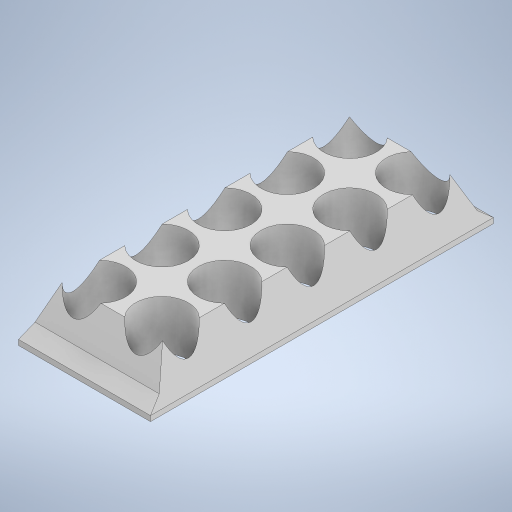
# Autodesk Inventor part: tray
Saved by Autodesk Inventor 2023 (Build 270158000, 158)
## iProperties
Created: 2023-01-16
Part Number: tray
Material: Generic
Document SubType Name: Modeling
Designer: Steven
Density: 1 g/cm^3
Appearance: Default
Author: Steven
Autodesk Inventor part; units mm, degrees
ref_plane "YZ Plane" through (0, 0, 0) normal (1, 0, 0) x (0, 1, 0)
ref_plane "XZ Plane" through (0, 0, 0) normal (0, 1, 0) x (-1, 0, 0)
ref_plane "XY Plane" through (0, 0, 0) normal (0, 0, 1) x (1, 0, 0)
sketch "Sketch1" plane through (0, 0, 0) normal (1, 0, 0) x (0, 1, 0)
  line L0 (0, 520) -> (0, 0)
  line L1 (144.6571, 260) -> (0, 260) construction
  line L2 (0, 0) -> (8, 0)
  line L3 (8, 0) -> (24.0697, 19.1511)
  line L4 (24.0697, 19.1511) -> (75, 42.9003)
  line L5 (0, 520) -> (8, 520)
  line L6 (8, 520) -> (24.0697, 500.8489)
  line L7 (24.0697, 500.8489) -> (75, 477.0997)
  line L8 (75, 477.0997) -> (75, 42.9003)
  dimension "d2" = 520
  dimension "d4" = 8
  dimension "d5" = 130
  dimension "d7" = 25
  dimension "d8" = 260
  dimension "d9" = 115
  dimension "d10" = 75
  constraints: 18 end point, 3 symmetric about line, 1 horizontal, 1 midpoint, 1 vertical
  measures "d2" distance of L0.start L0.end
  measures "d4" distance of L0.end L2.end
  measures "d5" angle of L2 L3
  measures "d7" distance of L2.end L3.end
  measures "d8" distance from line of L0.start L1
  measures "d9" angle of L4 L8
  measures "d10" distance from line of L0 L4.end
extrude "Extrusion1" add sketch "Sketch1" against normal blind 200
sketch "Sketch3" plane through (0, 0, 0) normal (0, 0, -1) x (-1, 0, 0)
  line L0 (0, 8) -> (0, 24.0697) projected
  line L1 (0, 8) -> (24.386, 75)
  line L2 (0, 75) -> (0, 8)
  line L3 (0, 24.0697) -> (0, 75) projected
  line L4 (100, 8) -> (100, 96) construction
  line L5 (200, 8) -> (175.614, 75)
  line L6 (200, 75) -> (200, 8)
  line L7 (0, 75) -> (24.386, 75)
  line L8 (0, 75) -> (200, 75) projected
  line L9 (175.614, 75) -> (200, 75)
  point P0 (0, 0)
  dimension "d13" = 20
  dimension "d14" = 20
  constraints: 14 end point, 2 horizontal, 1 collinear, 1 symmetric about line, 1 other
  measures "d13" angle of L2 L1
  measures "d14" angle of L6 L5
extrude "Extrusion2" cut sketch "Sketch3" against normal through all
sketch "Sketch4" plane through (-175.614, 75, 477.0997) normal (0, 1, 0) x (1, 0, 0)
  circle A0 centre (28.114, 27.0997) radius 40
  circle A1 centre (123.114, 27.0997) radius 40
  circle A2 centre (28.114, 122.0997) radius 40
  circle A3 centre (28.114, 217.0997) radius 40
  circle A4 centre (28.114, 312.0997) radius 40
  circle A5 centre (28.114, 407.0997) radius 40
  circle A6 centre (123.114, 407.0997) radius 40
  circle A7 centre (123.114, 312.0997) radius 40
  circle A8 centre (123.114, 217.0997) radius 40
  circle A9 centre (123.114, 122.0997) radius 40
  line L0 (-24.386, -42.9003) -> (-24.386, 477.0997) projected
  line L1 (175.614, 477.0997) -> (-24.386, 477.0997) projected
  line L2 (-24.386, 407.0997) -> (150.5812, 407.0997) construction
  line L3 (-24.386, 312.0997) -> (150.5812, 312.0997) construction
  line L4 (-24.386, 217.0997) -> (151.228, 217.0997) construction
  line L5 (151.228, 0) -> (151.228, 434.1994) construction
  line L6 (151.228, 122.0997) -> (-24.386, 122.0997) construction
  line L7 (-24.386, 27.0997) -> (151.228, 27.0997) construction
  line L8 (123.114, 434.1994) -> (123.114, 0) construction
  line L9 (151.228, 0) -> (0, 0) construction
  line L10 (151.228, 434.1994) -> (0, 434.1994) construction
  line L11 (28.114, 434.1994) -> (28.114, 0) construction
  dimension "d17" = 80
  dimension "d18" = 80
  dimension "d19" = 80
  dimension "d20" = 80
  dimension "d21" = 80
  dimension "d22" = 80
  dimension "d23" = 80
  dimension "d24" = 80
  dimension "d25" = 80
  dimension "d26" = 80
  dimension "d27" = 95
  dimension "d29" = 52.5
  dimension "d32" = 95
  dimension "d33" = 70
  dimension "d34" = 95
  dimension "d35" = 95
  dimension "d36" = 95
  constraints: 27 point on line, 14 end point, 10 centre point, 4 midpoint, 3 horizontal, 2 perpendicular, 1 parallel, 1 vertical
  measures "d17" diameter of A0
  measures "d18" diameter of A1
  measures "d19" diameter of A2
  measures "d20" diameter of A3
  measures "d21" diameter of A4
  measures "d22" diameter of A5
  measures "d23" diameter of A6
  measures "d24" diameter of A7
  measures "d25" diameter of A8
  measures "d26" diameter of A9
  measures "d27" distance of A6.centre A5.centre
  measures "d29" distance from line of L0 A5.centre
  measures "d32" distance between parallel lines of L2 L3
  measures "d33" distance between parallel lines of L1 L2
  measures "d34" distance between parallel lines of L3 L4
  measures "d35" distance between parallel lines of L4 L6
  measures "d36" distance between parallel lines of L7 L6
extrude "Extrusion3" cut sketch "Sketch4" against normal through all
body "Solid1"
